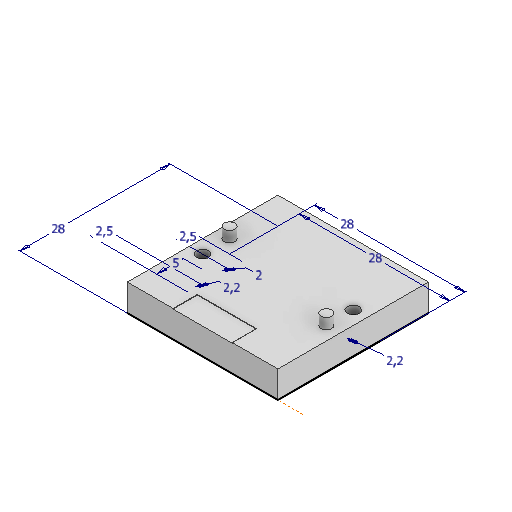
# Autodesk Inventor part: TracciaSopra
Saved by Autodesk Inventor 2025.4 (Build 294407000, 407)
## iProperties
Created: 2026-04-22
Part Number: TracciaSopra
Material: Generic
Document SubType Name: Modeling
Designer: gdira
Density: 1 g/cm^3
Appearance: Default
Author: gdira
Autodesk Inventor part; units mm, degrees
ref_plane "YZ Plane" through (0, 0, 0) normal (1, 0, 0) x (0, 1, 0)
ref_plane "XZ Plane" through (0, 0, 0) normal (0, 1, 0) x (-1, 0, 0)
ref_plane "XY Plane" through (0, 0, 0) normal (0, 0, 1) x (1, 0, 0)
sketch "Sketch1" plane through (0, 0, 0) normal (0, 1, 0) x (-1, 0, 0)
  line L0 (-15.486, -17.1716) -> (12.514, -17.1716)
  line L1 (12.514, 10.8284) -> (-15.486, 10.8284)
  line L2 (-20.486, 10.8284) -> (12.514, 10.8284) construction
  line L3 (-15.486, 5.8284) -> (-15.486, -12.1716)
  line L4 (12.514, 7.8284) -> (12.514, -12.1716)
  line L5 (12.514, -8.1716) -> (12.514, -3.1716)
  line L6 (7.514, -3.1716) -> (7.514, -8.1716)
  line L7 (7.514, -8.1716) -> (12.514, -8.1716)
  line L8 (12.514, 1.8284) -> (12.514, -3.1716)
  line L9 (7.514, -1.1716) -> (7.514, 1.8284)
  line L10 (7.514, 1.8284) -> (12.514, 1.8284)
  line L11 (12.514, -8.1716) -> (12.514, -3.1716)
  line L12 (12.514, -3.1716) -> (12.514, 1.8284)
  line L13 (12.514, 1.8284) -> (12.514, -3.1716)
  line L14 (12.514, -3.1716) -> (12.514, -8.1716)
  line L15 (12.514, -12.1716) -> (12.514, -17.1716)
  line L16 (12.514, 7.8284) -> (12.514, 10.8284)
  line L17 (-1.486, -17.1716) -> (-1.486, 10.8284)
  circle A0 centre (-12.986, -0.6716) radius 1
  line L18 (-10.486, 1.8284) -> (-15.486, 1.8284)
  line L19 (-15.486, 1.8284) -> (-15.486, -3.1716)
  line L20 (-15.486, -3.1716) -> (-15.486, 1.8284)
  line L21 (-15.486, 1.8284) -> (-15.486, -3.1716)
  line L22 (-10.486, -1.1716) -> (-10.486, 1.8284)
  circle A1 centre (-12.986, -5.6716) radius 1.1
  line L23 (-15.486, -8.1716) -> (-15.486, -3.1716)
  line L24 (-15.486, -8.1716) -> (-15.486, -3.1716)
  line L25 (-15.486, -3.1716) -> (-15.486, -8.1716)
  line L26 (-10.486, -3.1716) -> (-10.486, -8.1716)
  line L27 (-10.486, -8.1716) -> (-15.486, -8.1716)
  line L28 (-15.486, -12.1716) -> (-15.486, -17.1716)
  line L29 (-15.486, 7.8284) -> (-15.486, -12.1716)
  line L30 (-15.486, 10.8284) -> (-15.486, -17.1716)
  line L31 (10.014, -5.6716) -> (12.514, -5.6716)
  line L32 (10.014, -0.6716) -> (12.514, -0.6716)
  circle A2 centre (10.014, -5.6716) radius 1
  circle A3 centre (10.014, -0.6716) radius 1.1
  point P0 (0, 0)
  point P1 (10.014, -8.1716)
  point P2 (10.014, 1.8284)
  point P3 (-12.986, 1.8284)
  point P4 (-12.986, -8.1716)
  point P5 (12.514, 1.8284)
  point P6 (-15.486, 1.8284)
  point P7 (12.514, -8.1716)
  dimension "d0" = 5
  dimension "d1" = 2.5
  dimension "d2" = 2.5
  dimension "d3" = 2
  dimension "d4" = 2.2
  dimension "d5" = 2.2
  dimension "d6" = 28
  dimension "d7" = 28
  dimension "d19" = 28
  constraints: 66 end point, 14 symmetric about line, 5 midpoint, 4 centre point, 3 perpendicular, 3 point on line, 2 coincident, 1 horizontal, 1 parallel
  measures "d0" distance of L8.start L8.end
  measures "d1" distance of point (10.014, -8.172) L31.start
  measures "d2" distance of point (10.014, 1.828) L32.start
  measures "d3" diameter of A2
  measures "d4" diameter of A3
  measures "d5" diameter of A1
  measures "d6" distance between parallel lines of L23 L5
  measures "d7" distance between parallel lines of L1 L0
  measures "d19" distance of L0.start L15.end
extrude "Extrusion1" add sketch "Sketch1" along normal blind 5
extrude "Extrusion2" add sketch "Sketch1" along normal blind 7 contours A2 | A0
extrude "Extrusion3" add sketch "Sketch1" along normal blind 2.8 contours A3 | A1
sketch "Sketch2" plane through (0, 5, 0) normal (0, 1, 0) x (1, 0, 0)
  line L0 (-12.514, -10.8284) -> (15.486, -10.8284) projected
  line L1 (1.486, -10.8284) -> (6.986, -10.8284)
  line L2 (6.986, -10.8284) -> (6.986, -6.3284)
  line L3 (6.986, -6.3284) -> (-4.014, -6.3284)
  line L4 (-4.014, -6.3284) -> (-4.014, -10.8284)
  point P0 (0, 0)
  dimension "d14" = 5.5
  dimension "d15" = 4.5
  dimension "d16" = 11
  constraints: 8 end point, 3 perpendicular, 2 point on line, 1 midpoint
  measures "d14" distance of L1.start L1.end
  measures "d15" distance of L1.end L2.end
  measures "d16" distance of L2.end L3.end
extrude "Extrusion4" cut sketch "Sketch2" against normal blind 0.1
body "Solid1"
